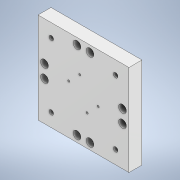
# Autodesk Inventor part: 土台
Saved by Autodesk Inventor 2021 (Build 250183000, 183)
## iProperties
Created: 2021-10-07
Part Number: 土台
Material: 一般
Document SubType Name: Modeling
Designer: ryusei
Density: 1 g/cm^3
Appearance: 滑らか - 白
Author: ryusei
Autodesk Inventor part; units mm, degrees
ref_plane "YZ Plane" through (0, 0, 0) normal (1, 0, 0) x (0, 1, 0)
ref_plane "XZ Plane" through (0, 0, 0) normal (0, 1, 0) x (-1, 0, 0)
ref_plane "XY Plane" through (0, 0, 0) normal (0, 0, 1) x (1, 0, 0)
sketch "スケッチ1" plane through (0, 0, 0) normal (0, 0, 1) x (1, 0, 0)
  line L0 (0, 0) -> (70, 0)
  line L1 (70, 0) -> (70, 70)
  line L2 (70, 70) -> (0, 70)
  line L3 (0, 70) -> (0, 0)
  dimension "d0" = 70
  dimension "d1" = 70
  constraints: 8 end point, 2 parallel, 1 horizontal, 1 perpendicular
  measures "d0" distance between parallel lines of L1 L3
  measures "d1" distance between parallel lines of L0 L2
extrude "押し出し1" add sketch "スケッチ1" along normal blind 10
sketch "スケッチ2" plane through (0, 0, 10) normal (0, 0, 1) x (1, 0, 0)
  line L0 (70, 70) -> (0, 70) projected
  line L1 (70, 0) -> (70, 70) projected
  line L2 (0, 0) -> (70, 0) projected
  line L3 (35, 70) -> (35, 0)
  point P0 (40, 65)
  point P1 (65, 40)
  point P2 (65, 30)
  point P3 (40, 5)
  point P4 (30, 65)
  point P5 (5, 40)
  point P6 (5, 30)
  point P7 (30, 5)
  dimension "d4" = 5
  dimension "d5" = 5
  dimension "d6" = 5
  dimension "d7" = 5
  dimension "d8" = 30
  dimension "d9" = 30
  dimension "d10" = 30
  dimension "d11" = 30
  constraints: 4 symmetric about line, 2 end point, 2 midpoint
  measures "d4" distance from line of L0 point (40, 65)
  measures "d5" distance from line of L1 point (65, 40)
  measures "d6" distance from line of L1 point (65, 30)
  measures "d7" distance from line of L2 point (40, 5)
  measures "d8" distance from line of L2 point (65, 30)
  measures "d9" distance from line of L1 point (40, 5)
  measures "d10" distance from line of L0 point (65, 40)
  measures "d11" distance from line of point (40, 65) L1
hole "穴1" at (40, 65, 10) at (65, 40, 10) at (65, 30, 10) at (40, 5, 10) at (30, 65, 10) at (5, 40, 10) at (5, 30, 10) at (30, 5, 10) direction (0, 0, -1) diameter 3.5 end through all counterbore diameter 6 counterbore depth 4
sketch "スケッチ10" plane through (0, 0, 10) normal (0, 0, 1) x (1, 0, 0)
  line L0 (0, 70) -> (0, 0) projected
  line L1 (70, 70) -> (0, 70) projected
  line L2 (0, 0) -> (70, 70)
  line L3 (70, 0) -> (70, 70) projected
  line L4 (70, 0) -> (0, 70)
  point P0 (10.2513, 59.7487)
  point P1 (59.7487, 10.2513)
  point P2 (10.2513, 10.2513)
  point P3 (59.7487, 59.7487)
  dimension "d41" = 70
  dimension "d42" = 70
  constraints: 4 end point, 2 point on line, 2 symmetric about line
  measures "d41" diameter of point (10.251, 59.749) L2
  measures "d42" diameter of point (10.251, 10.251) L4
hole "穴3" at (10.2513, 59.7487, 10) at (59.7487, 10.2513, 10) at (10.2513, 10.2513, 10) at (59.7487, 59.7487, 10) direction (0, 0, -1) diameter 3.5 end through all
sketch "スケッチ13" plane through (0, 0, 10) normal (0, 0, 1) x (1, 0, 0)
  line L0 (0, 70) -> (0, 0) projected
  line L1 (0, 0) -> (70, 0) projected
  line L2 (0, 70) -> (70, 0)
  line L3 (70, 70) -> (0, 70) projected
  line L4 (70, 70) -> (0, 0)
  point P0 (23.6863, 37.8284)
  point P1 (37.8284, 23.6863)
  point P2 (32.1716, 46.3137)
  point P3 (46.3137, 32.1716)
  dimension "d85" = 12
  dimension "d86" = 20
  dimension "d89" = 20
  dimension "d92" = 12
  constraints: 4 end point, 5 other
  measures "d85" diameter of point (23.686, 37.828) L2
  measures "d86" diameter of point (23.686, 37.828) L4
  measures "d89" distance of point (23.686, 37.828) point (37.828, 23.686)
  measures "d92" distance of point (23.686, 37.828) point (32.172, 46.314)
hole "穴6" at (23.6863, 37.8284, 10) at (37.8284, 23.6863, 10) at (32.1716, 46.3137, 10) at (46.3137, 32.1716, 10) direction (0, 0, -1) diameter 1.567 end through all thread size "M2x0.4" class "6H" standard "ISO Metric profile"
